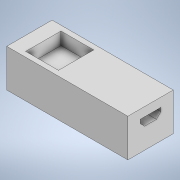
# Autodesk Inventor part: U2D2
Saved by Autodesk Inventor 2022 (Build 260153000, 153)
## iProperties
Created: 2021-09-20
Part Number: U2D2
Material: Generic
Document SubType Name: Modeling
Designer: kylem
Density: 1 g/cm^3
Appearance: Default
Author: kylem
Autodesk Inventor part; units mm, degrees
ref_plane "YZ Plane" through (0, 0, 0) normal (1, 0, 0) x (0, 1, 0)
ref_plane "XZ Plane" through (0, 0, 0) normal (0, 1, 0) x (-1, 0, 0)
ref_plane "XY Plane" through (0, 0, 0) normal (0, 0, 1) x (1, 0, 0)
sketch "Sketch1" plane through (0, 0, 0) normal (0, 1, 0) x (-1, 0, 0)
  line L0 (0, 0) -> (48, 0)
  line L1 (48, 0) -> (48, -18)
  line L2 (48, -18) -> (0, -18)
  line L3 (0, -18) -> (0, 0)
  dimension "d0" = 48
  dimension "d1" = 18
  constraints: 8 end point, 2 parallel, 1 horizontal, 1 perpendicular
  measures "d0" distance of L1.end L2.end
  measures "d1" distance of L0.end L1.end
extrude "Extrusion1" add sketch "Sketch1" along normal blind 15
sketch "Sketch2" plane through (0, 15, 0) normal (0, 1, 0) x (1, 0, 0)
  line L0 (-48, 18) -> (-48, 0) projected
  line L1 (-48, 0) -> (-42.5, 0)
  line L2 (-48, 0) -> (0, 0) projected
  line L3 (-42.5, 0) -> (-42.5, 2)
  line L4 (-42.5, 2) -> (-29.5, 2)
  line L5 (-29.5, 2) -> (-29.5, 16)
  line L6 (-42.5, 2) -> (-42.5, 16)
  line L7 (-42.5, 16) -> (-29.5, 16)
  dimension "d4" = 5.5
  dimension "d5" = 2
  dimension "d6" = 13
  dimension "d7" = 14
  constraints: 12 end point, 4 perpendicular, 1 point on line, 1 vertical
  measures "d4" distance of L0.end L1.end
  measures "d5" distance of L1.end L3.end
  measures "d6" distance of L3.end L4.end
  measures "d7" distance of L4.end L5.end
extrude "Extrusion2" cut sketch "Sketch2" against normal blind 5
sketch "Sketch3" plane through (0, 0, 0) normal (1, 0, 0) x (0, 0, -1)
  line L0 (0, 0) -> (0, 15)
  line L1 (0, 15) -> (18, 15)
  line L2 (16, 15) -> (2, 15) projected
  line L3 (9, 15) -> (9, 11.5)
  line L4 (9, 11.5) -> (13.1, 11.5)
  line L5 (13.1, 11.5) -> (4.9, 11.5)
  line L6 (4.9, 11.5) -> (4.9, 8.25)
  line L7 (4.9, 8.25) -> (13.1, 8.25)
  line L8 (13.1, 8.25) -> (13.1, 11.5)
  line L9 (16, 10) -> (2, 10) projected
  line L10 (4.9, 10) -> (7.1782, 7.7218)
  line L11 (4.9, 10) -> (8.1218, 10) construction
  line L12 (13.1, 10) -> (10.403, 7.303)
  line L13 (13.1, 10) -> (16.9142, 10) construction
  point P0 (11.35, 8.25)
  point P1 (6.65, 8.25)
  dimension "d10" = 18
  dimension "d11" = 3.5
  dimension "d12" = 4.1
  dimension "d13" = 8.2
  dimension "d14" = 3.25
  dimension "d15" = 45
  dimension "d16" = 135
  constraints: 24 end point, 5 point on line, 3 horizontal, 3 perpendicular, 2 equal length, 1 collinear, 1 midpoint, 1 vertical
  measures "d10" distance of L0.end L1.end
  measures "d11" distance of L3.start L3.end
  measures "d12" distance of L3.end L4.end
  measures "d13" distance of L4.end L5.end
  measures "d14" distance of L5.end L6.end
  measures "d15" angle of L10 L11
  measures "d16" angle of L12 L13
extrude "Extrusion3" cut sketch "Sketch3" against normal blind 5 contours L4 L8 L9 L6 L5 | L12 L7 L10 L9
body "Solid1"
